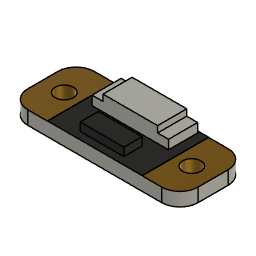
LED (Autodesk Fusion 360 design; units mm, degrees)
Autodesk Fusion 360 part; units mm, degrees
sketch "Sketch1" plane through (0, 0, 0) normal (0, 0, 1) x (1, 0, 0)
  line L0 (0, 0) -> (9.35, 0)
  line L1 (9.35, 0) -> (9.35, 3.65)
  line L2 (9.35, 3.65) -> (0, 3.65)
  line L3 (0, 3.65) -> (0, 0)
  line L4 (4.675, 3.65) -> (4.675, 0) construction
  line L5 (1.175, 1.825) -> (8.175, 1.825) construction
  circle A0 centre (1.175, 1.825) radius 0.5
  circle A1 centre (8.175, 1.825) radius 0.5
  dimension "d1" = 9.35
  dimension "d2" = 3.65
  dimension "d3" = 1
  dimension "d5" = 7
  constraint horizontal L0
  constraint vertical L1
  constraint horizontal L2
  constraint vertical L3
  constraint coincident L0.start L3.end
  constraint midpoint L2 L4.start
  constraint midpoint L0 L4.end
  constraint perpendicular L4 L5
  constraint midpoint L4 L5
  constraint coincident L5.start A0.centre
  constraint coincident L5.end A1.centre
  constraint equal A0 A1
  measures "d1" distance of L0.start L0.end
  measures "d2" distance of L0.start L2.end
  measures "d3" diameter of A0
  measures "d5" distance of L5.start L5.end
extrude "Extrude1" add sketch "Sketch1" along normal blind 0.75
fillet "Fillet1" radius 1 4 edges at (0, 0, 0.375) (0, 3.65, 0.375) (9.35, 3.65, 0.375) (9.35, 0, 0.375)
sketch "Sketch2" plane through (0, 0, 0.75) normal (0, 0, 1) x (-1, 0, 0)
  arc A0 (-8.35, 0) -> (-9.35, -1) centre (-8.35, -1) ccw
  line L0 (-9.35, -1) -> (-9.35, -2.65)
  arc A1 (-9.35, -2.65) -> (-8.35, -3.65) centre (-8.35, -2.65) ccw
  line L1 (-8.35, -3.65) -> (-1, -3.65)
  arc A2 (-1, -3.65) -> (0, -2.65) centre (-1, -2.65) ccw
  line L2 (0, -2.65) -> (0, -1)
  arc A3 (0, -1) -> (-1, 0) centre (-1, -1) ccw
  line L3 (-1, 0) -> (-8.35, 0)
  circle A4 centre (-1.175, -1.825) radius 0.5
  circle A5 centre (-8.175, -1.825) radius 0.5
  line L4 (-2.575, -3.55) -> (-6.775, -3.55)
  line L5 (-6.775, -3.55) -> (-6.775, -1.95)
  line L6 (-6.775, -1.95) -> (-2.575, -1.95)
  line L7 (-2.575, -1.95) -> (-2.575, -3.55)
  line L8 (-3.475, -1.4) -> (-5.875, -1.4)
  line L9 (-5.875, -1.4) -> (-5.875, -0.4)
  line L10 (-5.875, -0.4) -> (-3.475, -0.4)
  line L11 (-3.475, -0.4) -> (-3.475, -1.4)
  line L12 (-2.575, -2.75) -> (-6.775, -2.75) construction
  line L13 (-4.675, -3.65) -> (-4.675, -2.75) construction
  line L14 (-3.475, -0.9) -> (-5.875, -0.9) construction
  line L15 (-4.675, -0.9) -> (-4.675, -2.75) construction
  line L16 (-4.675, -0.9) -> (-4.675, 0) construction
  dimension "d10" = 1.6
  dimension "d11" = 4.2
  dimension "d12" = 0.1
  dimension "d13" = 1
  dimension "d14" = 2.4
  constraint horizontal L4
  constraint vertical L5
  constraint horizontal L6
  constraint vertical L7
  constraint horizontal L8
  constraint vertical L9
  constraint horizontal L10
  constraint vertical L11
  constraint midpoint L7 L12.start
  constraint midpoint L5 L12.end
  constraint midpoint L1 L13.start
  constraint midpoint L12 L13.end
  constraint midpoint L11 L14.start
  constraint midpoint L9 L14.end
  constraint midpoint L14 L15.start
  constraint midpoint L3 L16.end
  constraint vertical L13
  constraint vertical L15
  constraint equal L13 L16
  measures "d10" distance of L4.end L5.end
  measures "d11" distance of L4.start L4.end
  measures "d12" distance of L1 L4
  measures "d13" distance of L8.end L9.end
  measures "d14" distance of L9.end L10.end
extrude "Extrude2" add sketch "Sketch2" along normal blind 0.85 contours L4 L5 L6 L7
extrude "Extrude3" add sketch "Sketch2" along normal blind 0.45 contours L8 L9 L10 L11
sketch "Sketch3" plane through (0, 0, 1.6) normal (0, 0, 1) x (-1, 0, 0)
  line L0 (-2.575, -1.95) -> (-6.775, -1.95)
  line L1 (-6.775, -1.95) -> (-6.775, -3.55)
  line L2 (-6.775, -3.55) -> (-2.575, -3.55)
  line L3 (-2.575, -3.55) -> (-2.575, -1.95)
  line L4 (-3.175, -3.55) -> (-6.175, -3.55)
  line L5 (-6.175, -3.55) -> (-6.175, -1.95)
  line L6 (-6.175, -1.95) -> (-3.175, -1.95)
  line L7 (-3.175, -1.95) -> (-3.175, -3.55)
  line L8 (-4.675, -3.55) -> (-4.675, -1.95) construction
  line L9 (-2.575, -2.75) -> (-6.775, -2.75) construction
  dimension "d19" = 3
  constraint horizontal L4
  constraint vertical L5
  constraint horizontal L6
  constraint vertical L7
  constraint midpoint L4 L8.start
  constraint midpoint L6 L8.end
  constraint midpoint L3 L9.start
  constraint midpoint L1 L9.end
  constraint midpoint L8 L9
  constraint collinear L2 L4
  measures "d19" distance of L5 L7
extrude "Extrude4" cut sketch "Sketch3" against normal blind 0.35 contours L0 L2 L3 L7 | L0 L1 L2 L5
sketch "Sketch4" plane through (0, 0, 0.75) normal (0, 0, 1) x (-1, 0, 0)
  line L0 (-3.475, -0.4) -> (-3.475, -1.4)
  line L1 (-3.475, -1.4) -> (-5.875, -1.4)
  line L2 (-5.875, -1.4) -> (-5.875, -0.4)
  line L3 (-5.875, -0.4) -> (-3.475, -0.4)
  line L4 (-2.575, -1.95) -> (-2.575, -3.55)
  line L5 (-2.575, -3.55) -> (-6.775, -3.55)
  line L6 (-6.775, -3.55) -> (-6.775, -1.95)
  line L7 (-6.775, -1.95) -> (-2.575, -1.95)
  arc A0 (-8.35, 0) -> (-9.35, -1) centre (-8.35, -1) ccw
  line L8 (-9.35, -1) -> (-9.35, -2.65)
  arc A1 (-9.35, -2.65) -> (-8.35, -3.65) centre (-8.35, -2.65) ccw
  line L9 (-8.35, -3.65) -> (-1, -3.65)
  arc A2 (-1, -3.65) -> (0, -2.65) centre (-1, -2.65) ccw
  line L10 (0, -2.65) -> (0, -1)
  arc A3 (0, -1) -> (-1, 0) centre (-1, -1) ccw
  line L11 (-1, 0) -> (-8.35, 0)
  circle A4 centre (-1.175, -1.825) radius 0.5
  circle A5 centre (-8.175, -1.825) radius 0.5
  line L12 (-2.075, -3.65) -> (-7.275, -3.65)
  line L13 (-7.275, -3.65) -> (-7.275, 0)
  line L14 (-7.275, 0) -> (-2.075, 0)
  line L15 (-2.075, 0) -> (-2.075, -3.65)
  line L16 (-4.675, -3.65) -> (-4.675, 0) construction
  line L17 (0, -1.825) -> (-9.35, -1.825) construction
  dimension "d22" = 5.2
  constraint horizontal L12
  constraint vertical L13
  constraint horizontal L14
  constraint vertical L15
  constraint coincident L11 L13.end
  constraint coincident L9 L12.start
  constraint midpoint L12 L16.start
  constraint midpoint L14 L16.end
  constraint midpoint L10 L17.start
  constraint midpoint L8 L17.end
  constraint midpoint L16 L17
  measures "d22" distance of L13 L15
extrude "Extrude5" cut sketch "Sketch4" against normal blind 0.01 contours A0 L8 A1 L9 L11 L13 | L9 A2 L10 A3 L11 L15
sketch "Sketch5" plane through (0, 0, 0) normal (0, 0, 1) x (1, 0, 0)
move_body "Align1" bodies 1 to x (1, 0, 0) y (0, 1, 0) z (0, 0, 1) at (-4.675, -1.825, 0)
move_body "Move1" bodies 1 to x (1, 0, 0) y (0, 1, 0) z (0, 0, 1) at (0, 0, -0.37)
equation "d15 = 1.60 mm - 0.75 mm"
equation "d17 = 1.2 mm - 0.75 mm"
